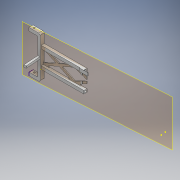
# Autodesk Inventor part: mtv_frame(BrakeInFront)2-6 - BACK
Saved by Autodesk Inventor 2018 (Build 220112000, 112)
## iProperties
Created: 2019-01-13
Part Number: mtv_frame(BrakeInFront)2-6 - BACK
Material: Generic
Document SubType Name: Modeling
Designer: aditya
Density: 1 g/cm^3
Appearance: Default
Author: aditya
## iProperties of the stored document mtv_frame(BrakeInFront)1-13_3DPrint.ipt
Created: 2019-01-14
Part Number: mtv_frame(BrakeInFront)1-13_3DPrint
Material: Generic
Document SubType Name: Modeling
Designer: aditya
Density: 1 g/cm^3
Appearance: Default
Author: aditya
Autodesk Inventor part; units mm, degrees
ref_plane "YZ Plane" through (0, 0, 0) normal (1, 0, 0) x (0, 1, 0)
ref_plane "XZ Plane" through (0, 0, 0) normal (0, 1, 0) x (-1, 0, 0)
ref_plane "XY Plane" through (0, 0, 0) normal (0, 0, 1) x (1, 0, 0)
sketch "Sketch1" plane through (0, 0, 0) normal (0, 1, 0) x (-1, 0, 0)
  line L0 (0, 0) -> (50, 0)
  line L1 (50, 0) -> (50, 50)
  line L2 (50, 50) -> (0, 50)
  line L3 (0, 50) -> (0, 0)
  line L4 (50, 50) -> (290, 50)
  line L5 (290, 50) -> (290, 42.5)
  line L6 (290, 42.5) -> (50, 42.5)
  line L7 (50, 42.5) -> (50, 50)
  line L8 (50, 0) -> (290, 0)
  line L9 (290, 0) -> (290, 7.5)
  line L10 (290, 7.5) -> (50, 7.5)
  line L11 (50, 7.5) -> (50, 0)
  dimension "d0" = 50
  dimension "d1" = 50
  dimension "d2" = 240
  dimension "d3" = 7.5
  dimension "d4" = 7.5
  constraints: 24 end point, 6 parallel, 3 horizontal, 3 perpendicular, 1 point on line
  measures "d0" distance of L2.end L1.end
  measures "d1" distance of L1.end L0.end
  measures "d2" distance of L5.end L6.end
  measures "d3" distance of L4.end L5.end
  measures "d4" distance of L9.end L8.end
extrude "Extrusion1" add sketch "Sketch1" along normal blind 7.5
sketch "Sketch2" plane through (0, 7.5, 0) normal (0, 1, 0) x (1, 0, 0)
  line L0 (0, -50) -> (0, 0) projected
  point P0 (0, -25)
  constraints: 1 midpoint
hole "Hole1" at (0, 7.5, 25) direction (0, -1, 0) diameter 6.35 end through all
sketch "Sketch3" plane through (0, 7.5, 0) normal (0, 1, 0) x (1, 0, 0)
  line L0 (-3.175, -50) -> (-3.175, 0) construction
  line L1 (-3.175, -50) -> (-28.175, -50) construction
  line L2 (-28.175, -50) -> (-28.175, 0) construction
  line L3 (-28.175, 0) -> (-3.175, 0) construction
  point P0 (0, 0)
  point P1 (-7.175, -4)
  point P2 (-24.175, -46)
  dimension "d14" = 25
  constraints: 8 end point, 2 perpendicular, 1 vertical
  measures "d14" distance of L0.start L1.end
hole "Hole2" at (-7.175, 7.5, 4) at (-24.175, 7.5, 46) direction (0, -1, 0) diameter 3.3 end through all
sketch "Sketch4" plane through (0, 7.5, 0) normal (0, 1, 0) x (1, 0, 0)
  arc A0 (0, -21.825) -> (0, -28.175) centre (0, -25) ccw construction
  line L0 (-3.175, -25) -> (-28.175, -25) construction
  line L1 (-3.175, -25) -> (21.825, -25) construction
  line L2 (-290, -50) -> (0, -50) construction
  line L3 (-28.175, -50) -> (-28.175, 0) construction
  line L4 (-50, -7.5) -> (-50, -42.5) construction
  line L5 (-50, -42.5) -> (-45, -42.5) construction
  line L6 (-45, -42.5) -> (-45, -32.5) construction
  line L7 (-45, -32.5) -> (-50, -32.5) construction
  line L8 (-50, -32.5) -> (-50, -42.5) construction
  line L9 (-45, -32.5) -> (-40, -32.5)
  line L10 (-40, -32.5) -> (-40, -42.5)
  line L11 (-40, -42.5) -> (-45, -42.5)
  line L12 (-45, -42.5) -> (-45, -32.5)
  point P0 (0, 0)
  dimension "d22" = 25
  dimension "d23" = 180
  dimension "d24" = 5
  dimension "d25" = 10
  dimension "d26" = 5
  constraints: 22 end point, 4 horizontal, 4 parallel, 2 perpendicular, 2 point on line, 1 collinear, 1 point on circle, 1 vertical
  measures "d22" distance of L0.start L0.end
  measures "d23" angle of L0 L1
  measures "d24" distance of L7.end L6.end
  measures "d25" distance of L6.end L5.end
  measures "d26" distance of L10.end L11.end
extrude "Extrusion2" add sketch "Sketch4" along normal blind 17.5
sketch "Sketch5" plane through (0, 7.5, 0) normal (0, 1, 0) x (1, 0, 0)
  line L0 (-85, -7.5) -> (-85, -42.5)
  line L1 (-127.5, -7.5) -> (-127.5, -42.5)
  line L2 (-92.5, -42.5) -> (-92.5, -7.5)
  line L3 (-135, -7.5) -> (-170, -7.5) construction
  line L4 (-170, -7.5) -> (-170, -42.5) construction
  line L5 (-170, -42.5) -> (-135, -42.5) construction
  line L6 (-135, -42.5) -> (-135, -7.5) construction
  line L7 (-177.5, -7.5) -> (-212.5, -7.5) construction
  line L8 (-212.5, -7.5) -> (-212.5, -42.5) construction
  line L9 (-212.5, -42.5) -> (-177.5, -42.5) construction
  line L10 (-177.5, -42.5) -> (-177.5, -7.5) construction
  line L11 (-220, -7.5) -> (-255, -7.5) construction
  line L12 (-255, -7.5) -> (-255, -42.5) construction
  line L13 (-255, -42.5) -> (-220, -42.5) construction
  line L14 (-220, -42.5) -> (-220, -7.5) construction
  line L15 (-85, -7.5) -> (-92.5, -7.5) construction
  line L16 (-92.5, -7.5) -> (-92.5, -42.5) construction
  line L17 (-92.5, -42.5) -> (-85, -42.5) construction
  line L18 (-85, -42.5) -> (-85, -7.5) construction
  line L19 (-127.5, -7.5) -> (-135, -7.5) construction
  line L20 (-135, -7.5) -> (-135, -42.5) construction
  line L21 (-135, -42.5) -> (-127.5, -42.5) construction
  line L22 (-127.5, -42.5) -> (-127.5, -7.5) construction
  line L23 (-170, -7.5) -> (-177.5, -7.5) construction
  line L24 (-177.5, -7.5) -> (-177.5, -42.5) construction
  line L25 (-177.5, -42.5) -> (-170, -42.5) construction
  line L26 (-170, -42.5) -> (-170, -7.5) construction
  line L27 (-212.5, -7.5) -> (-220, -7.5) construction
  line L28 (-220, -7.5) -> (-220, -42.5) construction
  line L29 (-220, -42.5) -> (-212.5, -42.5) construction
  line L30 (-212.5, -42.5) -> (-212.5, -7.5) construction
  line L31 (-220, -7.5) -> (-212.5, -7.5)
  line L32 (-212.5, -7.5) -> (-212.5, -42.5)
  line L33 (-212.5, -42.5) -> (-220, -42.5)
  line L34 (-220, -42.5) -> (-220, -7.5)
  line L35 (-177.5, -7.5) -> (-170, -7.5)
  line L36 (-170, -7.5) -> (-170, -42.5)
  line L37 (-170, -42.5) -> (-177.5, -42.5)
  line L38 (-177.5, -42.5) -> (-177.5, -7.5)
  line L39 (-135, -7.5) -> (-127.5, -7.5)
  line L40 (-127.5, -7.5) -> (-127.5, -42.5)
  line L41 (-127.5, -42.5) -> (-135, -42.5)
  line L42 (-135, -42.5) -> (-135, -7.5)
  line L43 (-92.5, -7.5) -> (-85, -7.5)
  line L44 (-85, -7.5) -> (-85, -42.5)
  line L45 (-85, -42.5) -> (-92.5, -42.5)
  line L46 (-92.5, -42.5) -> (-92.5, -7.5)
  point P0 (0, 0)
  point P1 (-50, -7.5)
  dimension "d30" = 35
  dimension "d31" = 35
  dimension "d32" = 35
  dimension "d33" = 35
  dimension "d34" = 35
  dimension "d35" = 35
  constraints: 94 end point, 23 parallel, 11 horizontal, 11 perpendicular
  measures "d30" distance of L2.start L1.end
  measures "d31" distance of L5.end L4.end
  measures "d32" distance of L4.end L3.end
  measures "d33" distance of L9.end L8.end
  measures "d34" distance of L8.end L7.end
  measures "d35" distance of L13.end L12.end
extrude "Extrusion3" add sketch "Sketch5" against normal blind 2
sketch "Sketch6" plane through (0, 7.5, 0) normal (0, 1, 0) x (1, 0, 0)
  line L0 (-290, 0) -> (-290, -7.5) projected
  line L1 (-290, -50) -> (0, -50) projected
  line L2 (-290, 0) -> (-280, 0)
  line L3 (-280, 0) -> (-280, -50)
  line L4 (-280, -50) -> (-290, -50)
  line L5 (-290, -50) -> (-290, 0)
  point P0 (0, 0)
  dimension "d38" = 10
  constraints: 8 end point, 2 parallel, 1 horizontal, 1 perpendicular, 1 point on line
  measures "d38" distance of L3.end L4.end
extrude "Extrusion4" cut sketch "Sketch6" against normal blind 7.5
sketch "Sketch7" plane through (-280, 7.5, 0) normal (-1, 0, 0) x (0, 0, 1)
  point P0 (0, -7.5)
sketch "Sketch8" plane through (-280, 7.5, 0) normal (-1, 0, 0) x (0, 0, 1)
  line L0 (-25, 0) -> (75, 0)
  line L1 (75, 0) -> (75, -7.5)
  line L2 (75, -7.5) -> (-25, -7.5)
  line L3 (-25, -7.5) -> (-25, 0)
  line L4 (-25, 0) -> (75, 0)
  line L5 (75, 0) -> (75, -10)
  line L6 (75, -10) -> (-25, -10)
  line L7 (-25, -10) -> (-25, 0)
  point P0 (0, -7.5)
  dimension "d41" = 100
  dimension "d42" = 10
  constraints: 16 end point, 4 parallel, 2 horizontal, 2 perpendicular
  measures "d41" distance of L1.end L2.end
  measures "d42" distance of L4.end L5.end
extrude "Extrusion5" add sketch "Sketch8" along normal blind 7.5
sketch "Sketch9" plane through (-287.5, 7.5, 0) normal (-1, 0, 0) x (0, 0, 1)
  line L0 (75, 0) -> (-25, 0) projected
  line L1 (-25, -10) -> (75, -10) projected
  line L2 (-25, 0) -> (-17.5, 0)
  line L3 (-17.5, 0) -> (-17.5, -10)
  line L4 (-17.5, -10) -> (-25, -10)
  line L5 (-25, -10) -> (-25, 0)
  line L6 (75, 0) -> (67.5, 0)
  line L7 (67.5, 0) -> (67.5, -10)
  line L8 (67.5, -10) -> (75, -10)
  line L9 (75, -10) -> (75, 0)
  point P0 (0, -7.5)
  dimension "d45" = 7.5
  dimension "d46" = 7.5
  constraints: 16 end point, 4 parallel, 2 horizontal, 2 perpendicular, 2 point on line
  measures "d45" distance of L3.end L4.end
  measures "d46" distance of L8.end L7.end
extrude "Extrusion6" add sketch "Sketch9" along normal blind 25 contours L9 L1 L7 L0 | L3 L1 L5 L0
sketch "Sketch10" plane through (-287.5, -2.5, -17.5) normal (0, 0, 1) x (1, 0, 0)
  line L0 (0, 0) -> (-25, 0) construction
  line L1 (0, 0) -> (-3, 0) construction
  line L2 (-3, 0) -> (-6.2, 0)
  line L3 (-6.2, 0) -> (-6.2, 2.1)
  line L4 (-6.2, 2.1) -> (-3, 2.1)
  line L5 (-3, 2.1) -> (-3, 0)
  line L6 (-6.2, 2.1) -> (-11.7, 2.1) construction
  line L7 (-11.7, 2.1) -> (-11.7, 5.4) construction
  point P0 (287.5, 2.5)
  dimension "d49" = 3
  dimension "d50" = 3.2
  dimension "d51" = 2.1
  dimension "d52" = 5.5
  dimension "d53" = 3.3
  constraints: 14 end point, 3 perpendicular, 2 point on line, 1 coincident, 1 horizontal, 1 vertical
  measures "d49" distance of L0.start L1.end
  measures "d50" distance of L1.end L2.end
  measures "d51" distance of L2.end L3.end
  measures "d52" distance of L3.end L6.end
  measures "d53" distance of L6.end L7.end
extrude "Extrusion7" add sketch "Sketch10" along normal blind 92.5
sketch "Sketch11" plane through (-287.5, -2.5, -17.5) normal (0, 0, 1) x (1, 0, 0)
  line L0 (-6.2, 2.1) -> (-3, 2.1) construction
  line L1 (-6.2, 2.1) -> (-11.7, 2.1) construction
  line L2 (-11.7, 2.1) -> (-11.7, 5.4) construction
  circle A0 centre (-11.7, 5.4) radius 2.125
  point P0 (287.5, 2.5)
  dimension "d56" = 5.5
  dimension "d57" = 3.3
  dimension "d58" = 4.25
  constraints: 4 end point, 1 centre point, 1 coincident, 1 horizontal, 1 perpendicular
  measures "d56" distance of L0.start L1.end
  measures "d57" distance of L1.end L2.end
  measures "d58" diameter of A0
extrude "Extrusion8" cut sketch "Sketch11" along normal mid plane 241
sketch "Sketch12" plane through (-287.5, -2.5, -17.5) normal (0, 0, 1) x (1, 0, 0)
  circle A0 centre (-11.7, 5.4) radius 2.125 construction
  line L0 (-11.7, 5.4) -> (-11.7, 0.96) construction
  line L1 (-11.7, 0.96) -> (-16.7, 0.96) construction
  line L2 (-6.2, 0) -> (-25, 0) projected
  line L3 (-16.7, 0.96) -> (-19.2, 0.96)
  line L4 (-19.2, 0.96) -> (-19.2, 0)
  line L5 (-19.2, 0) -> (-16.7, 0)
  line L6 (-16.7, 0) -> (-16.7, 0.96)
  point P0 (287.5, 2.5)
  dimension "d61" = 4.44
  dimension "d62" = 5
  dimension "d63" = 2.5
  constraints: 12 end point, 2 parallel, 2 perpendicular, 1 coincident, 1 horizontal, 1 point on line, 1 vertical
  measures "d61" distance of L0.start L0.end
  measures "d62" distance of L0.end L1.end
  measures "d63" distance of L5.end L4.end
extrude "Extrusion9" add sketch "Sketch12" along normal blind 91.25
sketch "Sketch13" plane through (-293.7, -0.4, -17.5) normal (0, 1, 0) x (1, 0, 0)
  line L0 (3.2, 0) -> (3.2, -85) construction
  line L1 (3.2, 0) -> (3.2, -30) construction
  line L2 (0, 0) -> (0, -85) construction
  line L3 (3.2, -30) -> (0, -30) construction
  line L4 (0, -30) -> (0, -36.35) construction
  line L5 (0, -36.35) -> (3.2, -36.35) construction
  line L6 (3.2, -36.35) -> (3.2, -30) construction
  line L7 (0, -30) -> (3.2, -30)
  line L8 (3.2, -30) -> (3.2, -36.35)
  line L9 (3.2, -36.35) -> (0, -36.35)
  line L10 (0, -36.35) -> (0, -30)
  point P0 (293.7, -17.5)
  dimension "d66" = 30
  dimension "d67" = 6.35
  constraints: 18 end point, 4 parallel, 2 horizontal, 2 perpendicular, 2 point on line
  measures "d66" distance of L0.start L1.end
  measures "d67" distance of L4.end L3.end
extrude "Extrusion10" add sketch "Sketch13" along normal blind 3.8
sketch "Sketch14" plane through (0, 7.5, 0) normal (0, 1, 0) x (1, 0, 0)
  line L0 (-287.5, 17.5) -> (-287.5, -67.5) projected
  line L1 (-287.5, 17.5) -> (-285, 17.5)
  line L2 (-285, 17.5) -> (-285, -67.5)
  line L3 (-285, -67.5) -> (-287.5, -67.5)
  line L4 (-287.5, -67.5) -> (-287.5, 17.5)
  point P0 (0, 0)
  dimension "d70" = 2.5
  constraints: 8 end point, 2 parallel, 1 horizontal, 1 perpendicular
  measures "d70" distance of L2.end L3.end
extrude "Extrusion11" cut sketch "Sketch14" against normal blind 14.55
sketch "Sketch15" plane through (0, 7.5, 0) normal (0, 1, 0) x (1, 0, 0)
  line L0 (-312.5, 17.5) -> (-312.5, 25) projected
  line L1 (-280, -75) -> (-312.5, -75) projected
  line L2 (-312.5, 25) -> (-306.6488, 25)
  line L3 (-306.6488, 25) -> (-306.6488, -75)
  line L4 (-306.6488, -75) -> (-312.5, -75)
  line L5 (-312.5, -75) -> (-312.5, 25)
  point P0 (0, 0)
  constraints: 8 end point, 2 parallel, 1 horizontal, 1 perpendicular, 1 point on line
extrude "Extrusion12" cut sketch "Sketch15" against normal blind 14.55
fillet "Fillet1" radius 0.1 1 edges at (-301.325, 2.9, -17.5)
fillet "Fillet2" radius 0.1 1 edges at (-301.325, 2.9, 67.5)
fillet "Fillet3" radius 3.25 1 edges at (-280, 2.5, 75)
fillet "Fillet4" radius 3.25 1 edges at (-285, 2.5, 67.5)
fillet "Fillet5" radius 3.25 1 edges at (-280, 2.5, -25)
fillet "Fillet6" radius 3.25 1 edges at (-285, 2.5, -17.5)
sketch "Sketch16" plane through (0, 7.5, 0) normal (0, 1, 0) x (1, 0, 0)
  line L0 (-220, -42.5) -> (-220, -7.5) construction
  line L1 (-220, -42.5) -> (-280, -42.5) construction
  line L2 (-220, -7.5) -> (-255, -7.5) construction
  line L3 (-255, -7.5) -> (-255, -42.5) construction
  line L4 (-255, -42.5) -> (-220, -42.5) construction
  line L5 (-220, -42.5) -> (-220, -7.5) construction
  line L6 (-280, -7.5) -> (-280, 0) projected
  line L7 (-280, -7.5) -> (-270, -7.5)
  line L8 (-270, -7.5) -> (-270, -42.5)
  line L9 (-270, -42.5) -> (-280, -42.5)
  line L10 (-280, -42.5) -> (-280, -7.5)
  point P0 (0, 0)
  dimension "d81" = 35
  dimension "d82" = 10
  constraints: 16 end point, 4 parallel, 2 horizontal, 2 perpendicular, 2 point on line
  measures "d81" distance of L4.end L3.end
  measures "d82" distance of L8.end L9.end
extrude "Extrusion13" add sketch "Sketch16" against normal blind 2
sketch "Sketch17" plane through (0, 7.5, 0) normal (0, 1, 0) x (1, 0, 0)
  point P0 (0, 0)
sketch "Sketch18" plane through (0, 7.5, 0) normal (0, 1, 0) x (1, 0, 0)
  line L0 (-270, -7.5) -> (-270, -42.5) construction
  line L1 (-285, -64.25) -> (-285, 14.25) construction
  line L2 (-280, -7.5) -> (-280, 0) construction
  line L3 (-270, -7.5) -> (-280, -7.5) construction
  line L4 (-275, -7.5) -> (-275, -42.5) construction
  line L5 (-50, -42.5) -> (-280, -42.5) construction
  circle A0 centre (-275, -12.5) radius 1.8 construction
  circle A1 centre (-275, -37.5) radius 1.8 construction
  circle A2 centre (-275, -12.5) radius 1.8
  circle A3 centre (-275, -37.5) radius 1.8
  point P0 (0, 0)
  dimension "d85" = 3.6
  dimension "d86" = 3.6
  constraints: 4 centre point, 4 end point, 3 point on line, 2 coincident, 2 concentric, 1 horizontal, 1 midpoint, 1 vertical
  measures "d85" diameter of A0
  measures "d86" diameter of A1
hole "Hole3" at (-275, 7.5, 12.5) at (-275, 7.5, 37.5) direction (0, -1, 0) diameter 3.3 depth 15 tip angle 118
sketch "Sketch19" plane through (0, 7.5, 0) normal (0, 1, 0) x (1, 0, 0)
  circle A0 centre (-275, -12.5) radius 1.65 construction
  line L0 (-275, -12.5) -> (-212.5, -12.5) construction
  line L1 (-212.5, -7.5) -> (-212.5, -42.5) construction
  circle A1 centre (-275, -37.5) radius 1.65 construction
  line L2 (-275, -37.5) -> (-212.5, -37.5) construction
  line L3 (-220, -42.5) -> (-220, -7.5) construction
  line L4 (-220, -12.5) -> (-212.5, -12.5) construction
  line L5 (-216.25, -12.5) -> (-216.25, -37.5) construction
  point P0 (0, 0)
  constraints: 8 end point, 4 point on line, 3 horizontal, 2 coincident, 1 midpoint, 1 perpendicular
hole "Hole4" at (-216.25, 7.5, 12.5) at (-216.25, 7.5, 37.5) direction (0, -1, 0) diameter 3.3 depth 15 tip angle 118
sketch "Sketch20" plane through (-45, 7.5, 32.5) normal (-1, 0, 0) x (0, 0, 1)
  line L0 (10, 17.5) -> (0, 17.5) construction
  line L1 (5, 17.5) -> (5, -0.1335) construction
  line L2 (10, 0) -> (10, 17.5) construction
  line L3 (10, 12.5) -> (5, 12.5) construction
  circle A0 centre (5, 12.5) radius 3
  point P0 (-32.5, -7.5)
  dimension "d101" = 6
  constraints: 4 end point, 2 coincident, 2 point on line, 1 centre point, 1 midpoint, 1 perpendicular, 1 vertical
  measures "d101" diameter of A0
extrude "Extrusion14" cut sketch "Sketch20" against normal blind 20
sketch "Sketch21" plane through (0, 7.5, 0) normal (0, 1, 0) x (1, 0, 0)
  line L0 (-306.6488, 17.5) -> (-306.6488, -67.5) projected
  line L1 (-306.6488, 17.5) -> (-288.25, 17.5) projected
  line L2 (-306.6488, -67.5) -> (-288.25, -67.5)
  line L3 (-288.25, -67.5) -> (-288.25, 17.5)
  line L4 (-288.25, 17.5) -> (-306.6488, 17.5)
  line L5 (-306.6488, 17.5) -> (-306.6488, -67.5)
  point P0 (0, 0)
  constraints: 8 end point, 2 parallel, 1 horizontal, 1 perpendicular
extrude "Extrusion15" cut sketch "Sketch21" against normal blind 10
sketch "Sketch22" plane through (0, 7.5, 0) normal (0, 1, 0) x (1, 0, 0)
  line L0 (-280, -50) -> (0, -50) projected
  line L1 (0, 0) -> (-280, 0) projected
  line L2 (-280, -50) -> (-270.5687, -50)
  line L3 (-270.5687, -50) -> (-270.5687, 0)
  line L4 (-270.5687, 0) -> (-280, 0)
  line L5 (-280, 0) -> (-280, -50)
  line L6 (-50, -42.5) -> (-280, -42.5) projected
  line L7 (-219.3019, -42.5) -> (-213.3073, -42.5)
  line L8 (-213.3073, -42.5) -> (-213.3073, -8.284)
  line L9 (-213.3073, -8.284) -> (-219.3019, -8.284)
  line L10 (-219.3019, -8.284) -> (-219.3019, -42.5)
  constraints: 16 end point, 4 parallel, 2 horizontal, 2 perpendicular, 2 point on line
extrude "Extrusion16" add sketch "Sketch22" against normal blind 2
sketch "Sketch23" plane through (-306.6488, -2.5, -25) normal (0, 0, -1) x (-1, 0, 0)
  circle A0 centre (-7.4488, 5.4) radius 2.125 projected
  circle A1 centre (-7.4488, 5.4) radius 2
  circle A2 centre (-7.4488, 5.4) radius 2.4429
  point P0 (-306.6488, 2.5)
  dimension "d108" = 4
  constraints: 2 centre point, 2 coincident
  measures "d108" diameter of A1
extrude "Extrusion17" add sketch "Sketch23" against normal blind 100 contours A0 | A2
sketch "Sketch24" plane through (0, 7.5, 0) normal (0, 1, 0) x (1, 0, 0)
  line L0 (-288.25, -67.5) -> (-306.6488, -67.5) projected
  arc A0 (-285, 14.25) -> (-288.25, 17.5) centre (-288.25, 14.25) ccw projected
  line L1 (-306.6488, -67.5) -> (-288.25, -67.5)
  line L2 (-288.25, -67.5) -> (-288.25, 17.5)
  line L3 (-288.25, 17.5) -> (-306.6488, 17.5)
  line L4 (-306.6488, 17.5) -> (-306.6488, -67.5)
  point P0 (0, 0)
  constraints: 8 end point, 2 parallel, 1 horizontal, 1 perpendicular
extrude "Extrusion18" cut sketch "Sketch24" against normal blind 100
sketch "Sketch25" plane through (0, 7.5, 0) normal (0, 1, 0) x (1, 0, 0)
  line L0 (-50, -42.5) -> (-280, -42.5) projected
  line L1 (-280, -7.5) -> (-50, -7.5) projected
  line L2 (-50, -42.5) -> (-55, -42.5)
  line L3 (-55, -42.5) -> (-55, -7.5)
  line L4 (-55, -7.5) -> (-50, -7.5)
  line L5 (-50, -7.5) -> (-50, -42.5)
  point P0 (0, 0)
  dimension "d113" = 5
  constraints: 8 end point, 2 parallel, 1 horizontal, 1 perpendicular, 1 point on line
  measures "d113" distance of L3.end L4.end
extrude "Extrusion19" add sketch "Sketch25" against normal blind 2
sketch "Sketch26" plane through (0, 7.5, 0) normal (0, 1, 0) x (1, 0, 0)
  line L0 (-55, -42.5) -> (-85, -42.5) construction
  line L1 (-55, -42.5) -> (-50, -42.5) construction
  line L2 (-55, -42.5) -> (-50, -42.5) construction
  line L3 (-50, -42.5) -> (-50, -7.5) construction
  line L4 (-50, -42.5) -> (-50, -7.5) construction
  circle A0 centre (-50, -37.5) radius 1.65 construction
  circle A1 centre (-50, -12.5) radius 1.65 construction
  circle A2 centre (-50, -37.5) radius 1.65
  circle A3 centre (-50, -12.5) radius 1.65
  line L5 (-50, -37.5) -> (-92.5, -37.5) construction
  line L6 (-92.5, -42.5) -> (-92.5, -7.5) construction
  line L7 (-50, -12.5) -> (-92.5, -12.5) construction
  line L8 (-92.5, -37.5) -> (-85, -37.5) construction
  line L9 (-85, -7.5) -> (-85, -42.5) construction
  line L10 (-88.75, -37.5) -> (-88.75, -12.5) construction
  circle A4 centre (-88.75, -37.5) radius 1.65
  circle A5 centre (-88.75, -12.5) radius 1.65
  point P0 (0, 0)
  dimension "d116" = 3.3
  dimension "d117" = 3.3
  dimension "d118" = 3.3
  dimension "d119" = 3.3
  constraints: 12 end point, 6 centre point, 5 point on line, 4 coincident, 2 concentric, 2 horizontal, 2 perpendicular, 1 collinear, 1 midpoint
  measures "d116" diameter of A0
  measures "d117" diameter of A1
  measures "d118" diameter of A4
  measures "d119" diameter of A5
extrude "Extrusion20" cut sketch "Sketch26" against normal blind 2
sketch "Sketch27" plane through (0, 5.5, 0) normal (0, -1, 0) x (1, 0, 0)
  line L0 (-50, 7.5) -> (-55, 7.5) projected
  line L1 (-55, 7.5) -> (-46.6169, 7.5)
  line L2 (-46.6169, 7.5) -> (-46.6169, 42.5)
  line L3 (-46.6169, 42.5) -> (-55, 42.5)
  line L4 (-55, 42.5) -> (-55, 7.5)
  point P0 (0, 0)
  constraints: 8 end point, 2 parallel, 1 horizontal, 1 perpendicular
extrude "Extrusion21" add sketch "Sketch27" along normal blind 5.5
sketch "Sketch28" plane through (0, 7.5, 0) normal (0, 1, 0) x (1, 0, 0)
  circle A0 centre (-50, -12.5) radius 1.65 projected
  circle A1 centre (-50, -37.5) radius 1.65 projected
  point P0 (0, 0)
  constraints: 2 coincident
hole "Hole5" at (-50, 7.5, 12.5) at (-50, 7.5, 37.5) direction (0, -1, 0) diameter 3.3 depth 8 tip angle 118
sketch "Sketch29" plane through (0, 7.5, 0) normal (0, 1, 0) x (1, 0, 0)
  circle A0 centre (-7.175, -4) radius 1.65 construction
  circle A1 centre (-24.175, -46) radius 1.65 construction
  line L0 (-7.175, -4) -> (-24.175, -46) construction
  line L1 (-7.175, -4) -> (-7.175, -46) construction
  line L2 (-7.175, -46) -> (-24.175, -46) construction
  line L3 (-7.175, -25) -> (-25.825, -25) construction
  line L4 (-25.825, -25) -> (-25.825, -46) construction
  line L5 (-16.5, -25) -> (-25.825, -25) construction
  line L6 (-24.175, -46) -> (-24.175, -25) construction
  line L7 (-15.675, -46) -> (-15.675, -4) construction
  line L8 (-40, -32.5) -> (-40, -42.5) construction
  line L9 (-40, -42.5) -> (-24.175, -42.5) construction
  line L10 (-24.175, -42.5) -> (-24.175, -46) construction
  line L11 (-15.675, -25) -> (-15.675, -46) construction
  line L12 (-15.675, -46) -> (-15.675, -4) construction
  circle A2 centre (-15.675, -46) radius 1.65 construction
  circle A3 centre (-15.675, -46) radius 1.65
  circle A4 centre (-15.675, -4) radius 1.65
  point P0 (0, 0)
  dimension "d131" = 42
  dimension "d132" = 17
  dimension "d133" = 21
  dimension "d135" = 8.5
  dimension "d136" = 15.825
  dimension "d137" = 3.5
  dimension "d138" = 21
  dimension "d139" = 3.3
  dimension "d140" = 3.3
  dimension "d141" = 3.3
  constraints: 24 end point, 4 collinear, 4 midpoint, 4 perpendicular, 3 centre point, 3 coincident, 3 point on line, 2 vertical, 1 horizontal, 1 horizontal alignment, 1 other
  measures "d131" distance of L0.start L1.end
  measures "d132" distance of L1.end L2.end
  measures "d133" distance of L3.end L4.end
  measures "d135" distance of L11.start L3.start
  measures "d136" distance of L8.end L9.end
  measures "d137" distance of L9.end L2.end
  measures "d138" distance of L11.start L7.start
  measures "d139" diameter of A2
  measures "d140" diameter of A3
  measures "d141" diameter of A4
extrude "Extrusion22" cut sketch "Sketch29" against normal blind 10
sketch "Sketch30" plane through (0, 7.5, 0) normal (0, 1, 0) x (1, 0, 0)
  circle A0 centre (-7.175, -4) radius 1.65 projected
  circle A1 centre (-7.175, -4) radius 2.1021
  circle A2 centre (-24.175, -46) radius 1.65 projected
  circle A3 centre (-24.175, -46) radius 2.9173
  point P0 (0, 0)
  constraints: 2 centre point, 2 coincident
extrude "Extrusion23" add sketch "Sketch30" against normal blind 7.5 contours A0 | A1 | A2 | A3
sketch "Sketch31" plane through (0, 25, 0) normal (0, 1, 0) x (1, 0, 0)
  line L0 (0, -50) -> (-177.5, -50)
  line L1 (-177.5, -50) -> (-177.5, 0)
  line L2 (-177.5, 0) -> (0, 0)
  line L3 (0, 0) -> (0, -50)
  constraints: 8 end point, 2 parallel, 1 horizontal, 1 perpendicular
extrude "Extrusion24" cut sketch "Sketch31" against normal blind 100
sketch "Sketch32" plane through (-177.5, 0, 42.5) normal (1, 0, 0) x (0, 0, -1)
  line L0 (56.75, 7.5) -> (-21.75, 7.5) construction
  line L1 (0, 0) -> (-7.5, 0) construction
  line L2 (0, 7.5) -> (-7.5, 0) construction
  line L3 (-7.5, 0) -> (-7.5, 7.5) construction
  line L4 (0, 0) -> (0, 5.5) construction
  line L5 (-7.5, 7.5) -> (0, 0) construction
  line L6 (35, 5.5) -> (35, 0) construction
  line L7 (35, 0) -> (42.5, 7.5) construction
  line L8 (35, 7.5) -> (42.5, 0) construction
  point P0 (38.75, 3.75)
  point P1 (-3.75, 3.75)
  constraints: 10 end point, 2 midpoint, 2 perpendicular, 2 point on line, 1 vertical
hole "Hole6" at (-177.5, 3.75, 3.75) at (-177.5, 3.75, 46.25) direction (-1, 0, 0) diameter 5 depth 15
sketch "Sketch33" plane through (-306.6488, -2.5, -25) normal (0, 0, -1) x (-1, 0, 0)
  circle A0 centre (-7.4488, 5.4) radius 2 projected
  circle A1 centre (-7.4488, 5.4) radius 2
  circle A2 centre (-7.4488, 5.4) radius 1.875
  point P0 (-306.6488, 2.5)
  dimension "d155" = 3.75
  constraints: 2 centre point, 2 coincident
  measures "d155" diameter of A2
extrude "Extrusion25" add sketch "Sketch33" against normal blind 100
sketch "Sketch34" plane through (0, 7.5, 0) normal (0, 1, 0) x (1, 0, 0)
  line L0 (-288.25, -67.5) -> (-306.6488, -67.5) projected
  line L1 (-306.6488, 17.5) -> (-288.25, 17.5) projected
  line L2 (-288.25, -67.5) -> (-306.6488, -67.5)
  line L3 (-306.6488, -67.5) -> (-306.6488, 17.5)
  line L4 (-306.6488, 17.5) -> (-288.25, 17.5)
  line L5 (-288.25, 17.5) -> (-288.25, -67.5)
  point P0 (0, 0)
  constraints: 8 end point, 2 parallel, 1 horizontal, 1 perpendicular
extrude "Extrusion26" cut sketch "Sketch34" against normal blind 100
sketch "Sketch35" plane through (-306.6488, 7.5, -25) normal (-1, 0, 0) x (0, 0, 1)
  line L0 (0, 0) -> (3.25, 0) projected
  line L1 (7.5, 0) -> (7.5, -10) projected
  line L2 (0, 0) -> (7.5, 0)
  line L3 (7.5, 0) -> (7.5, -10)
  line L4 (7.5, -10) -> (0, -10)
  line L5 (0, -10) -> (0, 0)
  point P0 (25, -7.5)
  constraints: 8 end point, 2 parallel, 1 horizontal, 1 perpendicular
ref_plane "Work Plane1" through (-306.6488, -2.5, -25) normal (0.0697565, -0.9975641, 0) x (0, 0, -1)
sketch "Sketch36" plane through (-306.6488, -2.5, -25) normal (0.0697565, -0.9975641, 0) x (0, 0, -1)
  point P0 (-25, 306.0762)
sketch "Sketch37" plane through (-306.6488, -2.5, -25) normal (0.0697565, -0.9975641, 0) x (0, 0, -1)
  line L0 (-51.6055, 16.5999) -> (-51.6055, 26.5838) construction
  line L1 (-51.6055, 26.5838) -> (-48.3945, 26.5838) construction
  line L2 (-48.3945, 26.5838) -> (-48.3945, 16.5999) construction
  line L3 (-48.3945, 16.5999) -> (-51.6055, 16.5999) construction
  line L4 (-51.6055, 16.5999) -> (-48.3945, 26.5838) construction
  line L5 (-51.6055, 26.5838) -> (-48.3945, 16.5999) construction
  line L6 (-48.3945, 26.5838) -> (-51.6055, 21.596) construction
  line L7 (-89.25, 21.596) -> (-10.75, 21.596) construction
  line L8 (-48.3945, 21.5919) -> (-51.6055, 26.5838) construction
  line L9 (-52.5, 21.5879) -> (-47.5, 21.5879)
  line L10 (-47.5, 21.5879) -> (-47.5, 26.5879)
  line L11 (-47.5, 26.5879) -> (-52.5, 26.5879)
  line L12 (-52.5, 26.5879) -> (-52.5, 21.5879)
  line L13 (-52.5, 21.5879) -> (-47.5, 26.5879) construction
  line L14 (-47.5, 21.5879) -> (-52.5, 26.5879) construction
  point P0 (-25, 306.0762)
  point P1 (-50, 21.5919)
  point P2 (-50, 24.0879)
  dimension "d161" = 5
  dimension "d162" = 5
  constraints: 28 end point, 6 midpoint, 4 parallel, 2 perpendicular, 2 point on line, 1 horizontal
  measures "d161" distance of L11.end L10.end
  measures "d162" distance of L10.end L9.end
extrude "Extrusion27" add sketch "Sketch37" along normal blind 37.5
sketch "Sketch38" plane through (-285.1135, -0.9941, 22.5) normal (-0.9975641, -0.0697565, 0) x (0, 0, 1)
  circle A0 centre (2.5, -36) radius 0.55
  point P0 (-22.5, -18.8968)
  dimension "d165" = 1.1
  constraints: 1 centre point
  measures "d165" diameter of A0
extrude "Extrusion28" cut sketch "Sketch38" against normal blind 37.5
fillet "Fillet7" radius 0.2 1 edges at (-282.6022, -36.9064, 24.45)
sketch "Sketch39" plane through (0, 5.5, 0) normal (0, -1, 0) x (1, 0, 0)
  line L0 (-280, 27.5) -> (-280, 22.5) construction
  line L1 (-280, 25) -> (-177.5, 25) construction
  line L2 (-177.5, 26.5) -> (-280, 26.5)
  line L3 (-280, 26.5) -> (-280, 23.5)
  line L4 (-280, 23.5) -> (-177.5, 23.5)
  line L5 (-177.5, 23.5) -> (-177.5, 26.5)
  line L6 (-177.5, 26.5) -> (-280, 23.5) construction
  line L7 (-280, 26.5) -> (-177.5, 23.5) construction
  point P0 (0, 0)
  point P1 (-228.75, 25)
  dimension "d169" = 3
  constraints: 14 end point, 4 midpoint, 2 horizontal, 2 parallel, 1 perpendicular, 1 point on line
  measures "d169" distance of L3.end L2.end
extrude "Extrusion29" add sketch "Sketch39" along normal blind 5.5
sketch "Sketch40" plane through (0, 7.5, 0) normal (0, 1, 0) x (1, 0, 0)
  line L0 (-177.5, -42.5) -> (-177.5, -50) projected
  line L1 (-270, -7.5) -> (-280, -7.5) projected
  line L2 (-177.5, -42.5) -> (-280, -42.5)
  line L3 (-280, -42.5) -> (-280, -7.5)
  line L4 (-280, -7.5) -> (-177.5, -7.5)
  line L5 (-177.5, -7.5) -> (-177.5, -42.5)
  point P0 (0, 0)
  constraints: 8 end point, 2 parallel, 1 horizontal, 1 perpendicular
extrude "Extrusion30" cut sketch "Sketch40" against normal blind 10
sketch "Sketch41" plane through (0, 7.5, 0) normal (0, 1, 0) x (1, 0, 0)
  line L0 (-280, -42.5) -> (-280, -7.5) construction
  line L1 (-280, -7.5) -> (-177.5, -7.5) construction
  line L2 (-280, -42.5) -> (-205.276, -42.5) construction
  line L3 (-205.276, -42.5) -> (-205.276, -7.5) construction
  line L4 (-205.276, -7.5) -> (-280, -7.5) construction
  line L5 (-280, -7.5) -> (-280, -42.5) construction
  line L6 (-205.276, -7.5) -> (-130.552, -7.5) construction
  line L7 (-130.552, -7.5) -> (-130.552, -42.5) construction
  line L8 (-130.552, -42.5) -> (-205.276, -42.5) construction
  line L9 (-205.276, -42.5) -> (-205.276, -7.5) construction
  line L10 (-280, -42.5) -> (-205.276, -7.5) construction
  line L11 (-280, -7.5) -> (-280, 0) construction
  line L12 (-280, -7.5) -> (-205.276, -42.5) construction
  line L13 (-205.276, -42.5) -> (-130.552, -7.5) construction
  line L14 (-205.276, -7.5) -> (-130.552, -42.5) construction
  line L15 (-202.8571, -9.1276) -> (-280.2981, -45.4003)
  line L16 (-280.2981, -45.4003) -> (-282.4189, -40.8724)
  line L17 (-282.4189, -40.8724) -> (-204.9779, -4.5997)
  line L18 (-204.9779, -4.5997) -> (-202.8571, -9.1276)
  line L19 (-202.8571, -9.1276) -> (-282.4189, -40.8724) construction
  line L20 (-280.2981, -45.4003) -> (-204.9779, -4.5997) construction
  line L21 (-280.627, -5.219) -> (-202.6026, -40.219)
  line L22 (-202.6026, -40.219) -> (-204.649, -44.781)
  line L23 (-204.649, -44.781) -> (-282.6734, -9.781)
  line L24 (-282.6734, -9.781) -> (-280.627, -5.219)
  line L25 (-280.627, -5.219) -> (-204.649, -44.781) construction
  line L26 (-202.6026, -40.219) -> (-282.6734, -9.781) construction
  line L27 (-129.925, -5.219) -> (-207.9494, -40.219)
  line L28 (-207.9494, -40.219) -> (-205.903, -44.781)
  line L29 (-205.903, -44.781) -> (-127.8786, -9.781)
  line L30 (-127.8786, -9.781) -> (-129.925, -5.219)
  line L31 (-129.925, -5.219) -> (-205.903, -44.781) construction
  line L32 (-207.9494, -40.219) -> (-127.8786, -9.781) construction
  line L33 (-207.6949, -9.1276) -> (-130.2539, -45.4003)
  line L34 (-130.2539, -45.4003) -> (-128.1331, -40.8724)
  line L35 (-128.1331, -40.8724) -> (-205.5741, -4.5997)
  line L36 (-205.5741, -4.5997) -> (-207.6949, -9.1276)
  line L37 (-207.6949, -9.1276) -> (-128.1331, -40.8724) construction
  line L38 (-130.2539, -45.4003) -> (-205.5741, -4.5997) construction
  point P0 (0, 0)
  point P1 (-242.638, -25)
  point P2 (-242.638, -25)
  point P3 (-167.914, -25)
  dimension "d174" = 74.724
  dimension "d175" = 74.724
  dimension "d176" = 85.515
  dimension "d177" = 5
  dimension "d178" = 85.515
  dimension "d179" = 5
  dimension "d180" = 85.515
  dimension "d181" = 5
  dimension "d182" = 85.515
  dimension "d183" = 5
  constraints: 72 end point, 12 parallel, 11 midpoint, 6 perpendicular, 2 horizontal, 2 point on line
  measures "d174" distance of L4.end L3.end
  measures "d175" distance of L7.end L8.end
  measures "d176" distance of L15.start L15.end
  measures "d177" distance of L15.end L16.end
  measures "d178" distance of L21.start L21.end
  measures "d179" distance of L21.end L22.end
  measures "d180" distance of L27.start L27.end
  measures "d181" distance of L28.end L27.end
  measures "d182" distance of L33.start L33.end
  measures "d183" distance of L34.end L33.end
extrude "Extrusion31" add sketch "Sketch41" against normal blind 2 contours L18 L35 L27 L33 L15 | L15 L33 L36 L17 L35 L18 | L15 L21 L17 L36 L33 | L35 L17 L18 | L21 L27 L28 L23 L15 | L15 L23 L17 L21 | L33 L29 L22 L21 L27 | L27 L35 L29 L33 | L27 L30 L29 L35 | L17 L36 L35 | L15 L16 L17 L23 | L17 L23 L24 L21 | L21 L22 L29 L23 L28 L27 | L29 L35 L34 L33 | L23 L29 L28 | L22 L23 L29
sketch "Sketch42" plane through (0, 7.5, 0) normal (0, 1, 0) x (1, 0, 0)
  line L0 (-280, -50) -> (-177.5, -50) construction
  line L1 (-177.5, -50) -> (-167.5, -50) construction
  line L2 (-167.5, -50) -> (-167.5, 0) construction
  line L3 (-167.5, 0) -> (-177.5, 0) construction
  line L4 (-177.5, 0) -> (-177.5, -50) construction
  line L5 (-167.5, 0) -> (-117.2384, 0)
  line L6 (-117.2384, 0) -> (-117.2384, -74.5393)
  line L7 (-117.2384, -74.5393) -> (-167.5, -74.5393)
  line L8 (-167.5, -74.5393) -> (-167.5, 0)
  point P0 (0, 0)
  dimension "d186" = 10
  constraints: 16 end point, 4 parallel, 2 horizontal, 2 perpendicular
  measures "d186" distance of L3.end L2.end
extrude "Extrusion32" cut sketch "Sketch42" against normal blind 2
sketch "Sketch43" plane through (0, 7.5, 0) normal (0, 1, 0) x (1, 0, 0)
  point P0 (0, 0)
fillet "Fillet8" radius 2 15 edges at (-205.276, 6.5, 10.2606) (-205.276, 6.5, 39.0197) (-242.6605, 6.5, 22.2499) (-173.9127, 6.5, 24.9509) (-248.6367, 6.5, 25.0491) (-242.6155, 6.5, 27.7501) (-236.6393, 6.5, 24.9509) (-275.542, 6.5, 7.5) (-274.1061, 6.5, 42.5) (-200.818, 6.5, 42.5) (-199.3821, 6.5, 7.5) (-209.734, 6.5, 42.5) (-211.1699, 6.5, 7.5) (-280, 6.5, 10.9803) (-280, 6.5, 39.7394)
sketch "Sketch44" plane through (0, 7.5, 0) normal (0, 1, 0) x (1, 0, 0)
  line L0 (-177.5, -7.5) -> (-177.5, 0) projected
  line L1 (-177.5, 0) -> (-165.9736, 0)
  line L2 (-165.9736, 0) -> (-165.9736, -50.6569)
  line L3 (-165.9736, -50.6569) -> (-177.5, -50.6569)
  line L4 (-177.5, -50.6569) -> (-177.5, 0)
  point P0 (0, 0)
  constraints: 8 end point, 2 parallel, 1 horizontal, 1 perpendicular
extrude "Extrusion33" cut sketch "Sketch44" against normal blind 1
sketch "Sketch45" plane through (0, 7.5, 0) normal (0, 1, 0) x (1, 0, 0)
  line L0 (-177.5, -23.3205) -> (-177.5, -17.7494) projected
  line L1 (-177.5, -17.7494) -> (-164.6881, -17.7494)
  line L2 (-164.6881, -17.7494) -> (-164.6881, -33.2033)
  line L3 (-164.6881, -33.2033) -> (-177.5, -33.2033)
  line L4 (-177.5, -33.2033) -> (-177.5, -17.7494)
  point P0 (0, 0)
  constraints: 8 end point, 2 parallel, 1 horizontal, 1 perpendicular
extrude "Extrusion34" cut sketch "Sketch45" against normal blind 2
sketch "Sketch46" plane through (0, 5.5, 0) normal (0, -1, 0) x (1, 0, 0)
  line L0 (-177.5, 42.5) -> (-191.4729, 42.5) projected
  line L1 (-190.397, 7.5) -> (-177.5, 7.5) projected
  line L2 (-177.5, 42.5) -> (-187.5, 42.5)
  line L3 (-187.5, 42.5) -> (-187.5, 7.5)
  line L4 (-187.5, 7.5) -> (-177.5, 7.5)
  line L5 (-177.5, 7.5) -> (-177.5, 42.5)
  point P0 (0, 0)
  dimension "d194" = 10
  constraints: 8 end point, 2 parallel, 1 horizontal, 1 perpendicular, 1 point on line
  measures "d194" distance of L4.end L3.end
extrude "Extrusion35" cut sketch "Sketch46" against normal blind 1
sketch "Sketch47" plane through (0, 0, 0) normal (0, -1, 0) x (1, 0, 0)
  line L0 (-280, 50) -> (-177.5, 50) projected
  line L1 (-167.5, 42.5) -> (-187.5, 42.5)
  line L2 (-187.5, 42.5) -> (-187.5, 50)
  line L3 (-187.5, 50) -> (-167.5, 50)
  line L4 (-167.5, 50) -> (-167.5, 42.5)
  line L5 (-177.5, 48.75) -> (-177.5, 43.75) projected
  line L6 (-167.5, 42.5) -> (-187.5, 50) construction
  line L7 (-187.5, 42.5) -> (-167.5, 50) construction
  point P0 (0, 0)
  point P1 (-177.5, 46.25)
  dimension "d197" = 20
  constraints: 12 end point, 3 midpoint, 2 parallel, 1 horizontal, 1 perpendicular, 1 point on line
  measures "d197" distance of L2.end L3.end
extrude "Extrusion36" add sketch "Sketch47" along normal blind 1
body "Solid1"
